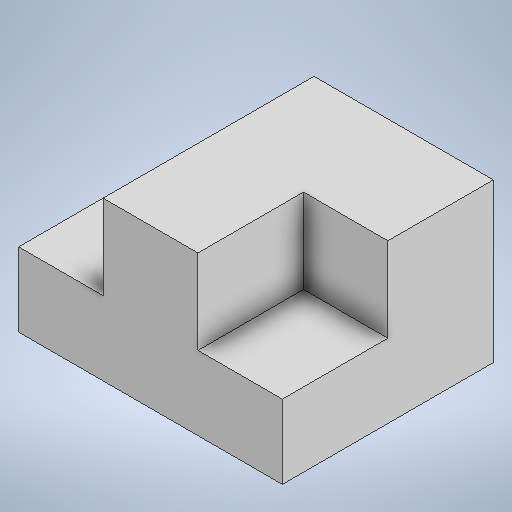
# Autodesk Inventor part: 視圖範例
Saved by Autodesk Inventor 2025 (Build 290162010, 162A)
## iProperties
Created: 2024-10-26
Part Number: 視圖範例
Material: 一般
Document SubType Name: Modeling
Designer: owner
Density: 1 g/cm^3
Appearance: 預設
Author: owner
Autodesk Inventor part; units mm, degrees
ref_plane "YZ Plane" through (0, 0, 0) normal (1, 0, 0) x (0, 1, 0)
ref_plane "XZ Plane" through (0, 0, 0) normal (0, 1, 0) x (-1, 0, 0)
ref_plane "XY Plane" through (0, 0, 0) normal (0, 0, 1) x (1, 0, 0)
sketch "草圖1" plane through (0, 0, 0) normal (0, 0, 1) x (1, 0, 0)
  line L0 (-12.5, -7.5) -> (12.5, -7.5)
  line L1 (12.5, -7.5) -> (12.5, 7.5)
  line L2 (12.5, 7.5) -> (-12.5, 7.5)
  line L3 (-12.5, 7.5) -> (-12.5, -7.5)
  line L4 (-12.5, -7.5) -> (12.5, 7.5) construction
  line L5 (12.5, -7.5) -> (-12.5, 7.5) construction
  point P0 (0, 0)
  dimension "d0" = 25
  dimension "d1" = 15
  constraints: 12 end point, 2 midpoint, 2 parallel, 1 horizontal, 1 perpendicular
  measures "d0" distance of L1.end L2.end
  measures "d1" distance of L0.end L1.end
extrude "擠出1" add sketch "草圖1" along normal mid plane 20
sketch "草圖2" plane through (0, 0, 10) normal (0, 0, 1) x (1, 0, 0)
  line L0 (12.5, 7.5) -> (-12.5, 7.5) projected
  line L1 (-12.5, 7.5) -> (-4.5, 7.5)
  line L2 (-4.5, 7.5) -> (-4.5, -0.5)
  line L3 (-4.5, -0.5) -> (-12.5, -0.5)
  line L4 (-12.5, -0.5) -> (-12.5, 7.5)
  line L5 (12.5, 7.5) -> (4.5, 7.5)
  line L6 (4.5, 7.5) -> (4.5, -0.5)
  line L7 (4.5, -0.5) -> (12.5, -0.5)
  line L8 (12.5, -0.5) -> (12.5, 7.5)
  point P0 (0, 0)
  point P1 (-4.5, 7.5)
  dimension "d4" = 8
  dimension "d5" = 8
  dimension "d6" = 8
  constraints: 16 end point, 4 parallel, 2 horizontal, 2 perpendicular, 1 point on line
  measures "d4" distance of L2.end L3.end
  measures "d5" distance of L6.end L7.end
  measures "d6" distance of L5.end L6.end
extrude "擠出2" cut sketch "草圖2" against normal blind 10 contours L8 L7 L6 L0
extrude "擠出3" cut sketch "草圖2" against normal blind 20 contours L2 L3 L4 L0
